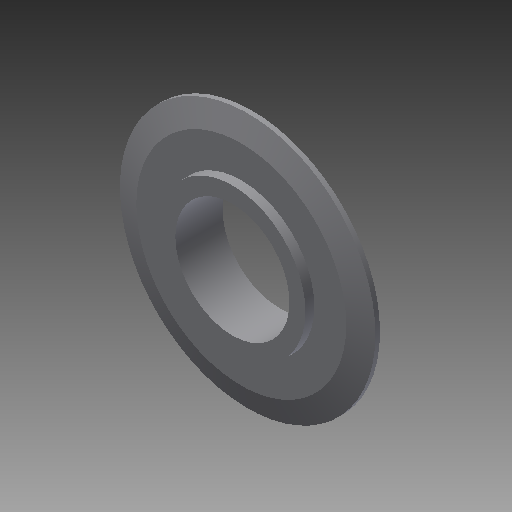
# Autodesk Inventor part: KL-SL-023-KMB-601-PT
Saved by Autodesk Inventor 2018 (Build 220112000, 112)
## iProperties
Created: 2015-08-01
Part Number: KL-SL-023-KMB-601-PT
Material: 一般
Document SubType Name: Modeling
Designer: Eric
Density: 1 g/cm^3
Appearance: 預設
Author: Eric
Autodesk Inventor part; units mm, degrees
ref_plane "YZ Plane" through (0, 0, 0) normal (1, 0, 0) x (0, 1, 0)
ref_plane "XZ Plane" through (0, 0, 0) normal (0, 1, 0) x (-1, 0, 0)
ref_plane "XY Plane" through (0, 0, 0) normal (0, 0, 1) x (1, 0, 0)
sketch "草圖1" plane through (0, 0, 0) normal (0, 0, 1) x (1, 0, 0)
  circle A0 centre (0, 0) radius 16
  constraints: 1 centre point
extrude "擠出1" add sketch "草圖1" along normal blind 6
sketch "草圖2" plane through (0, 0, 6) normal (0, 0, 1) x (1, 0, 0)
  circle A0 centre (0, 0) radius 28
  constraints: 1 centre point
extrude "擠出2" add sketch "草圖2" along normal blind 2.4
sketch "草圖3" plane through (0, 0, 8.4) normal (0, 0, 1) x (1, 0, 0)
  circle A0 centre (0, 0) radius 16
  constraints: 1 centre point
extrude "擠出3" add sketch "草圖3" along normal blind 1.95
hole "孔1" at (0, 0, 10.35) direction (0, 0, -1) diameter 25 end through all
chamfer "倒角1" distance 1.4 distance2 5 1 edges at (-28, 0, 8.4) measured on face at (27.9092, -2.2531, 7.6)
